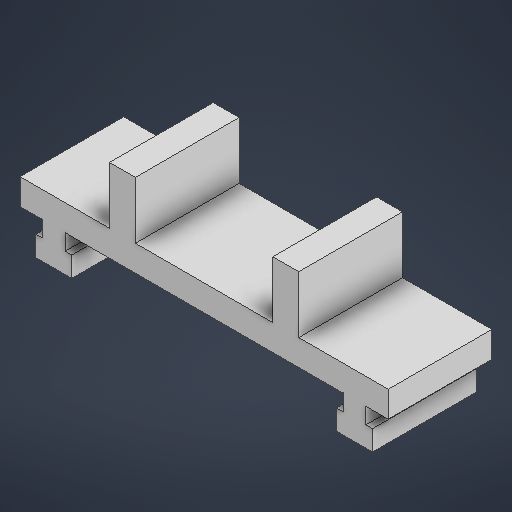
# Autodesk Inventor part: UnitreeGO2_railmount
Saved by Autodesk Inventor 2026.1 (Build 301233000, 233)
## iProperties
Created: 2026-01-16
Part Number: UnitreeGO2_railmount
Material: Generic
Document SubType Name: Modeling
Designer: aimot
Density: 1 g/cm^3
Appearance: Default
Author: aimot
Autodesk Inventor part; units mm, degrees
ref_plane "YZ Plane" through (0, 0, 0) normal (1, 0, 0) x (0, 1, 0)
ref_plane "XZ Plane" through (0, 0, 0) normal (0, 1, 0) x (-1, 0, 0)
ref_plane "XY Plane" through (0, 0, 0) normal (0, 0, 1) x (1, 0, 0)
sketch "Sketch2" plane through (0, 0, 0) normal (0, 0, 1) x (1, 0, 0)
  line L0 (-32.475, -3.1) -> (-25.525, -3.1)
  line L1 (-25.525, -3.1) -> (-25.525, -7)
  line L2 (-25.525, -7) -> (-32.475, -7)
  line L3 (-32.475, -7) -> (-32.475, -3.1)
  line L4 (-31.2, 0) -> (-26.8, 0)
  line L5 (-26.8, 0) -> (-26.8, -3.1)
  line L6 (-26.8, -3.1) -> (-31.2, -3.1)
  line L7 (-31.2, -3.1) -> (-31.2, 0)
  line L8 (-35.5, 0) -> (0, 0)
  line L9 (0, 5) -> (-35.5, 5)
  line L10 (-35.5, 5) -> (-35.5, 0)
  line L11 (-29, 6.5254) -> (-29, -10.3092) construction
  line L12 (0, -15.571) -> (0, 21.2618) construction
  line L13 (32.475, -3.1) -> (25.525, -3.1)
  line L14 (25.525, -3.1) -> (25.525, -7)
  line L15 (25.525, -7) -> (32.475, -7)
  line L16 (32.475, -7) -> (32.475, -3.1)
  line L17 (31.2, 0) -> (26.8, 0)
  line L18 (26.8, 0) -> (26.8, -3.1)
  line L19 (26.8, -3.1) -> (31.2, -3.1)
  line L20 (31.2, -3.1) -> (31.2, 0)
  line L21 (35.5, 0) -> (0, 0)
  line L22 (0, 5) -> (35.5, 5)
  line L23 (35.5, 5) -> (35.5, 0)
  line L24 (29, 6.5254) -> (29, -10.3092) construction
  line L25 (-49.7, 0) -> (49.7, 0) construction
  line L26 (-18.25, 5) -> (-18.25, 16)
  line L27 (-18.25, 16) -> (-13.25, 16)
  line L28 (-13.25, 16) -> (-13.25, 5)
  line L29 (18.25, 5) -> (18.25, 16)
  line L30 (18.25, 16) -> (13.25, 16)
  line L31 (13.25, 16) -> (13.25, 5)
  point P0 (13.25, 5)
  dimension "d1" = 4.4
  dimension "d2" = 6.95
  dimension "d3" = 3.9
  dimension "d4" = 5
  dimension "d5" = 58
  dimension "d6" = 7
  dimension "d7" = 13
  dimension "d10" = 5
  dimension "d15" = 26.5
  dimension "d16" = 11
  constraints: 60 end point, 15 symmetric about line, 7 parallel, 7 point on line, 4 horizontal, 4 perpendicular, 1 collinear, 2 other
  measures "d1" distance between parallel lines of L5 L7
  measures "d2" distance between parallel lines of L1 L3
  measures "d3" distance between parallel lines of L2 L0
  measures "d4" distance between parallel lines of L9 L8
  measures "d5" distance between parallel lines of L24 L11
  measures "d6" distance between parallel lines of L8 L2
  measures "d7" diameter of L10 L11
  measures "d10" distance between parallel lines of L28 L26
  measures "d15" distance between parallel lines of L31 L28
  measures "d16" distance between parallel lines of L9 L27
extrude "Extrusion1" add sketch "Sketch2" along normal blind 20
body "Solid1"
